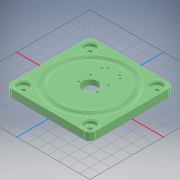
# Autodesk Inventor part: 000.005.001.001 - Основание
Saved by Autodesk Inventor 2022 (Build 260153000, 153)
## iProperties
Created: 2022-11-17
Part Number: 000.005.001.001 - Основание
Material: Пластик АБС
Document SubType Name: Modeling
Designer: Petrov Ivan
Density: 1.06 g/cm^3
Appearance: Гладкий — темный травянисто-зеленый
Author: Petrov Ivan
Autodesk Inventor part; units mm, degrees
ref_plane "YZ Plane" through (0, 0, 0) normal (1, 0, 0) x (0, 1, 0)
ref_plane "XZ Plane" through (0, 0, 0) normal (0, 1, 0) x (-1, 0, 0)
ref_plane "XY Plane" through (0, 0, 0) normal (0, 0, 1) x (1, 0, 0)
sketch "Эскиз1" plane through (0, 0, 0) normal (0, 1, 0) x (-1, 0, 0)
  line L0 (-80, 80) -> (80, 80)
  line L1 (80, 80) -> (80, -80)
  line L2 (80, -80) -> (-80, -80)
  line L3 (-80, -80) -> (-80, 80)
  line L4 (-80, 80) -> (80, -80) construction
  line L5 (80, 80) -> (-80, -80) construction
  point P0 (0, 0)
  dimension "d0" = 160
  dimension "d1" = 160
  constraints: 12 end point, 2 midpoint, 2 parallel, 1 horizontal, 1 perpendicular
  measures "d0" distance of L1.end L2.end
  measures "d1" distance of L0.end L1.end
extrude "Выдавливание1" add sketch "Эскиз1" along normal blind 15
sketch "Эскиз2" plane through (0, 15, 0) normal (0, 1, 0) x (1, 0, 0)
  circle A0 centre (0, 0) radius 70 construction
  circle A1 centre (0, 0) radius 60 construction
  circle A2 centre (0, 0) radius 65
  dimension "d4" = 140
  dimension "d5" = 120
  dimension "d6" = 130
  constraints: 3 centre point, 3 coincident
  measures "d4" diameter of A0
  measures "d5" diameter of A1
  measures "d6" diameter of A2
sketch "Эскиз3" plane through (0, 0, 0) normal (0, 0, 1) x (1, 0, 0)
  line L0 (65, 15) -> (-65, 15) projected
  circle A0 centre (-65, 15) radius 5.15
  point P0 (0, 0)
  dimension "d7" = 10.3
  constraints: 1 centre point, 1 coincident
  measures "d7" diameter of A0
sweep "Сдвиг1" cut profiles "Эскиз3" path "Эскиз2"
fillet "Сопряжение1" radius 3 2 edges at (-70.15, 15, 0) (-59.85, 15, 0)
sketch "Эскиз4" plane through (0, 15, 0) normal (0, 1, 0) x (1, 0, 0)
  circle A0 centre (0, 0) radius 15
  dimension "d11" = 30
  constraints: 1 centre point, 1 coincident
  measures "d11" diameter of A0
extrude "Выдавливание2" cut sketch "Эскиз4" against normal through all
fillet "Сопряжение2" radius 10 4 edges at (80, 7.5, 80) (-80, 7.5, 80) (-80, 7.5, -80) (80, 7.5, -80)
sketch "Эскиз5" plane through (0, 15, 0) normal (0, 1, 0) x (1, 0, 0)
  line L0 (0, 0) -> (-63.6396, -63.6396) construction
  circle A0 centre (-63.6396, -63.6396) radius 4.25
  line L1 (0, 0) -> (0, -19.7371) construction
  dimension "d15" = 90
  dimension "d16" = 8.5
  dimension "d17" = 45
  constraints: 4 end point, 1 centre point, 1 coincident, 1 vertical
  measures "d15" distance of L0.start L0.end
  measures "d16" diameter of A0
  measures "d17" angle of L1 L0
extrude "Выдавливание3" cut sketch "Эскиз5" against normal through all
sketch "Эскиз6" plane through (0, 15, 0) normal (0, 1, 0) x (1, 0, 0)
  circle A0 centre (-63.6396, -63.6396) radius 4.25 projected
  circle A1 centre (-63.6396, -63.6396) radius 11.5
  point P0 (0, 0)
  dimension "d20" = 23
  constraints: 1 centre point, 1 coincident
  measures "d20" diameter of A1
extrude "Выдавливание4" cut sketch "Эскиз6" against normal blind 8
chamfer "Фаска1" distance 2 angle 45 1 edges at (-75.1396, 15, 63.6396)
pattern_circular "Круговой массив1" count 4 over 360 about axis through (0, 15, 0) along (0, -1, 0) of "Выдавливание3", "Выдавливание4", "Фаска1"
sketch "Эскиз7" plane through (0, 0, 0) normal (0, -1, 0) x (1, 0, 0)
  arc A0 (20.1, 4.5766) -> (19.5808, 6.2636) centre (17.1, 4.5766) ccw
  line L0 (19.5808, 6.2636) -> (15.5953, 12.1246)
  arc A1 (15.5953, 12.1246) -> (13.9414, 13) centre (13.9414, 11) ccw
  line L1 (13, 13) -> (13.9414, 13)
  arc A2 (14.5, 11.5) -> (13, 13) centre (13, 11.5) ccw
  line L2 (14.5, -41.5) -> (14.5, 11.5)
  arc A3 (13.5, -42.5) -> (14.5, -41.5) centre (13.5, -41.5) ccw
  line L3 (-13.5, -42.5) -> (13.5, -42.5)
  arc A4 (-14.5, -41.5) -> (-13.5, -42.5) centre (-13.5, -41.5) ccw
  line L4 (-14.5, 11.5) -> (-14.5, -41.5)
  arc A5 (-13, 13) -> (-14.5, 11.5) centre (-13, 11.5) ccw
  line L5 (-13.9414, 13) -> (-13, 13)
  arc A6 (-13.9414, 13) -> (-15.5953, 12.1246) centre (-13.9414, 11) ccw
  line L6 (-15.5953, 12.1246) -> (-19.5808, 6.2636)
  arc A7 (-19.5808, 6.2636) -> (-20.1, 4.5766) centre (-17.1, 4.5766) ccw
  line L7 (-20.1, 4.5766) -> (-20.1, -39.6766)
  arc A8 (-20.1, -39.6766) -> (-19.5808, -41.3636) centre (-17.1, -39.6766) ccw
  line L8 (-19.5808, -41.3636) -> (-15.8929, -46.7869)
  arc A9 (-15.8929, -46.7869) -> (-13.4121, -48.1) centre (-13.4121, -45.1) ccw
  line L9 (-13.4121, -48.1) -> (13.4121, -48.1)
  arc A10 (13.4121, -48.1) -> (15.8929, -46.7869) centre (13.4121, -45.1) ccw
  line L10 (15.8929, -46.7869) -> (19.5808, -41.3636)
  arc A11 (19.5808, -41.3636) -> (20.1, -39.6766) centre (17.1, -39.6766) ccw
  line L11 (20.1, -39.6766) -> (20.1, 4.5766)
  circle A12 centre (-17.3, 4) radius 1.35
  circle A13 centre (-17.3, -18) radius 1.35
  circle A14 centre (-11, -45.3) radius 1.35
  circle A15 centre (17.3, 4) radius 1.35
  circle A16 centre (17.3, -18) radius 1.35
  circle A17 centre (11, -45.3) radius 1.35
  circle A18 centre (-17.3, -40) radius 1.35
  circle A19 centre (17.3, -40) radius 1.35
  line L12 (13, 13) -> (-13, 13)
  point P0 (0, 0)
  point P1 (0, 0)
  constraints: 26 end point, 24 point on circle, 20 centre point
extrude "Выдавливание5" cut sketch "Эскиз7" against normal blind 4 contours A2 L2 A3 L3 A4 L4 A5 L12
sketch "Эскиз8" plane through (0, 0, 0) normal (0, -1, 0) x (1, 0, 0)
  arc A0 (20.1, 4.5766) -> (19.5808, 6.2636) centre (17.1, 4.5766) ccw
  line L0 (19.5808, 6.2636) -> (15.5953, 12.1246)
  arc A1 (15.5953, 12.1246) -> (13.9414, 13) centre (13.9414, 11) ccw
  line L1 (13, 13) -> (13.9414, 13)
  arc A2 (14.5, 11.5) -> (13, 13) centre (13, 11.5) ccw
  line L2 (14.5, -41.5) -> (14.5, 11.5)
  arc A3 (13.5, -42.5) -> (14.5, -41.5) centre (13.5, -41.5) ccw
  line L3 (-13.5, -42.5) -> (13.5, -42.5)
  arc A4 (-14.5, -41.5) -> (-13.5, -42.5) centre (-13.5, -41.5) ccw
  line L4 (-14.5, 11.5) -> (-14.5, -41.5)
  arc A5 (-13, 13) -> (-14.5, 11.5) centre (-13, 11.5) ccw
  line L5 (-13.9414, 13) -> (-13, 13)
  arc A6 (-13.9414, 13) -> (-15.5953, 12.1246) centre (-13.9414, 11) ccw
  line L6 (-15.5953, 12.1246) -> (-19.5808, 6.2636)
  arc A7 (-19.5808, 6.2636) -> (-20.1, 4.5766) centre (-17.1, 4.5766) ccw
  line L7 (-20.1, 4.5766) -> (-20.1, -39.6766)
  arc A8 (-20.1, -39.6766) -> (-19.5808, -41.3636) centre (-17.1, -39.6766) ccw
  line L8 (-19.5808, -41.3636) -> (-15.8929, -46.7869)
  arc A9 (-15.8929, -46.7869) -> (-13.4121, -48.1) centre (-13.4121, -45.1) ccw
  line L9 (-13.4121, -48.1) -> (13.4121, -48.1)
  arc A10 (13.4121, -48.1) -> (15.8929, -46.7869) centre (13.4121, -45.1) ccw
  line L10 (15.8929, -46.7869) -> (19.5808, -41.3636)
  arc A11 (19.5808, -41.3636) -> (20.1, -39.6766) centre (17.1, -39.6766) ccw
  line L11 (20.1, -39.6766) -> (20.1, 4.5766)
  circle A12 centre (-17.3, 4) radius 1.35
  circle A13 centre (-17.3, -18) radius 1.35
  circle A14 centre (-11, -45.3) radius 1.35
  circle A15 centre (17.3, 4) radius 1.35
  circle A16 centre (17.3, -18) radius 1.35
  circle A17 centre (11, -45.3) radius 1.35
  circle A18 centre (-17.3, -40) radius 1.35
  circle A19 centre (17.3, -40) radius 1.35
  line L12 (13, 13) -> (-13, 13)
  point P0 (0, 0)
  point P1 (0, 0)
  point P2 (0, 0)
  constraints: 26 end point, 24 point on circle, 20 centre point
extrude "Выдавливание6" cut sketch "Эскиз8" against normal through all contours A12 | A13 | A14 | A15 | A16 | A17 | A18 | A19
move faces "Перенос1" translate (0, 0, -0.5) faces at (-4.5, 1.3333, -42.5)
sketch "Эскиз9" plane through (0, 15, 0) normal (0, 1, 0) x (1, 0, 0)
  circle A0 centre (17.3, 40) radius 1.35 projected
  circle A1 centre (11, 45.3) radius 1.35 projected
  circle A2 centre (-11, 45.3) radius 1.35 projected
  circle A3 centre (-17.3, 40) radius 1.35 projected
  circle A4 centre (-17.3, 18) radius 1.35 projected
  circle A5 centre (17.3, 18) radius 1.35 projected
  circle A6 centre (-17.3, -4) radius 1.35 projected
  circle A7 centre (17.3, -4) radius 1.35 projected
  point P0 (0, 0)
  constraints: 8 coincident
sketch "Эскиз10" plane through (0, 15, 0) normal (0, 1, 0) x (1, 0, 0)
  circle A0 centre (17.3, -4) radius 1.35 projected
  circle A1 centre (17.3, -4) radius 2.5
  point P0 (0, 0)
  dimension "d36" = 5
  constraints: 1 centre point, 1 coincident
  measures "d36" diameter of A1
extrude "Выдавливание7" cut sketch "Эскиз10" against normal blind 10 contours A0 | A1
pattern_sketch "Массив по эскизу1" of "Выдавливание7" from (17.3, 15, 4) copies at (17.3, 15, -40) at (11, 15, -45.3) at (-11, 15, -45.3) at (-17.3, 15, -40) at (-17.3, 15, -18) at (17.3, 15, -18) at (-17.3, 15, 4)
equation "\"d6\" = 0.5 * d5 + 0.5 * d4"
